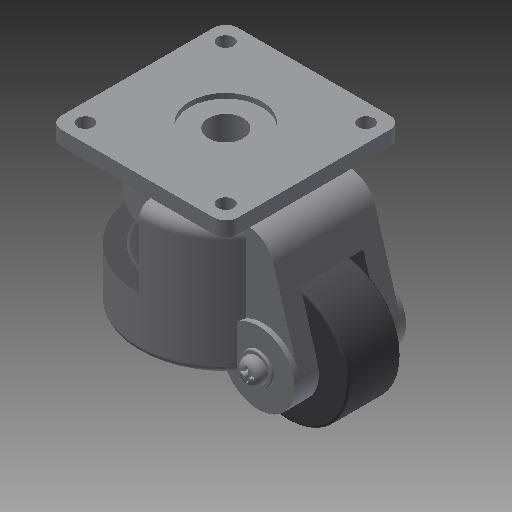
# Autodesk Inventor part: MayTec 1.45.80200.073_Locking castor 200kg, with plate
Saved by Autodesk Inventor 2018 (Build 220112000, 112)
## iProperties
Category: PARTsolutions
Company: MAYTEC
Created: 2012-11-13
Part Number: MayTec 1.45.80200.073_Locking castor 200kg, with plate
Catalog Web Link: www.cadenas.de
Description: Locking castor 200kg, with plate-Locking castor 200kg, with plate
Vendor: MAYTEC
Document SubType Name: Modeling
Designer: PARTuser1
Manufacturer: MAYTEC
Density: 1 g/cm^3
Material: Generic
Appearance: RGB(175.94999939203154,175.94999939203154,175.94999939203154)
PSOL_IDENT_0: {\\10.0.0.242\data_v9\23d-libs\maytec\maytec_3d\einbauzubehoer\rollen\feststell-rollen\1.45.80200.07
PSOL_IDENT_1: 3.prj},276 {VTYP=3D},{NB=MayTec 1.45.80200.073_Locking castor 200kg, with plate},{LINA=MayTec 1.45.8
PSOL_IDENT_2: 0200.073_Locking castor 200kg, with plate},{NN=Locking castor 200kg, with plate},{DATE=14.09.2010 08
PSOL_IDENT_3: :34:49},{GEOMDATE=28.01.2010 00:00:00},{VERSION=},{LINEID=10},{LINESUBID=-1},{WBVAR=}  {NB=MayTec 1.
PSOL_IDENT_4: 45.80200.073_Locking castor 200kg, with plate},{LINA=MayTec 1.45.80200.073_Locking castor 200kg, wit
PSOL_IDENT_5: h plate},{KT=DUMMY},{PARTNR=1.45.80200.073},{DESCRIPTION=Feststell-Rolle 200kg, mit Platte},{D=50.0}
PSOL_IDENT_6: ,{XTRANS=Locking castor 200kg, with plate}
CNS_NT: Locking castor 200kg, with plate
CNS_NB: MayTec 1.45.80200.073_Locking castor 200kg, with plate
CNS_NBSYN: MayTec $PARTNR._$XTRANS.
CNS_LINA: MayTec 1.45.80200.073_Locking castor 200kg, with plate
CNS_PARTNR: 1.45.80200.073
CNS_DESCRIPTION: Feststell-Rolle 200kg, mit Platte
CNS_D: 50.0
CNS_XTRANS: Locking castor 200kg, with plate
SUPPLIER: MAYTEC
ARTICLENO: MayTec 1.45.80200.073_Locking castor 200kg, with plate
BOMINFO: MayTec 1.45.80200.073_Locking castor 200kg, with plate
CREATOR: CADENAS GmbH
Title: MayTec 1.45.80200.073_Locking castor 200kg, with plate
Author: Cadenas PARTsolutions
Comments: Locking castor 200kg, with plate
Autodesk Inventor part; units mm, degrees
sketch "Sketch_2" plane through (0, 0, 0) normal (0, 1, 0) x (-1, 0, 0)
  line L0 (36.5, -31.5) -> (36.5, 31.5)
  arc A0 (36.5, 31.5) -> (31.5, 36.5) centre (31.5, 31.5) ccw
  line L1 (31.5, 36.5) -> (-31.5, 36.5)
  arc A1 (-31.5, 36.5) -> (-36.5, 31.5) centre (-31.5, 31.5) ccw
  line L2 (-36.5, 31.5) -> (-36.5, -31.5)
  arc A2 (-36.5, -31.5) -> (-31.5, -36.5) centre (-31.5, -31.5) ccw
  line L3 (-31.5, -36.5) -> (31.5, -36.5)
  arc A3 (31.5, -36.5) -> (36.5, -31.5) centre (31.5, -31.5) ccw
  circle A4 centre (-29, 29) radius 3.25
  circle A5 centre (-29, -29) radius 3.25
  circle A6 centre (29, 29) radius 3.25
  circle A7 centre (29, -29) radius 3.25
  constraints: 8 centre point, 8 end point, 8 point on circle
sketch "Sketch_1" plane through (0, 0, 0) normal (0, 0, 1) x (1, 0, 0)
  line L0 (0, -72) -> (0, -6)
  line L1 (0, -6) -> (29, -6)
  arc A0 (29, -6) -> (27.5, -7) centre (29.4232, -8.2598) ccw
  line L2 (27.5, -7) -> (17.5, -7)
  line L3 (17.5, -7) -> (17.5, -8)
  line L4 (17.5, -8) -> (28.5, -8)
  arc A1 (29, -8.5) -> (28.5, -8) centre (28.5, -8.5) ccw
  line L5 (29, -8.5) -> (29, -9.5)
  arc A2 (29, -9.5) -> (31, -11.5) centre (31, -9.5) ccw
  arc A3 (36, -16.5) -> (31, -11.5) centre (31, -16.5) ccw
  line L6 (36, -16.5) -> (36, -62)
  arc A4 (33, -65) -> (36, -62) centre (33, -62) ccw
  line L7 (33, -65) -> (30, -65)
  arc A5 (29, -64) -> (30, -65) centre (30, -64) ccw
  line L8 (29, -64) -> (29, -41)
  line L9 (29, -41) -> (28, -41)
  line L10 (28, -41) -> (28, -59)
  arc A6 (27.6154, -60.9231) -> (28, -59) centre (23, -59) ccw
  line L11 (27.6154, -60.9231) -> (24.2821, -68.9231)
  arc A7 (19.6667, -72) -> (24.2821, -68.9231) centre (19.6667, -67) ccw
  line L12 (19.6667, -72) -> (0, -72)
  line L13 (0, -72) -> (0, -6)
  constraints: 28 end point, 16 point on circle, 8 centre point
sketch "Sketch_3" plane through (0, 0, 0) normal (0, 0, 1) x (1, 0, 0)
  line L0 (14.7107, -52.434) -> (23.2335, -52.434)
  line L1 (23.2335, -52.434) -> (23.2335, -65)
  arc A0 (23.2335, -65) -> (50.8593, -53.6628) centre (36.5, -58) ccw
  line L2 (50.8593, -53.6628) -> (40.6951, -19.4721)
  arc A1 (40.6951, -19.4721) -> (31, -11.5) centre (29.9412, -22.669) ccw
  line L3 (31, -11.5) -> (14.7107, -11.5)
  line L4 (14.7107, -11.5) -> (14.7107, -52.434)
  constraints: 10 end point, 4 point on circle, 2 centre point
extrude "Extrusion1" add sketch "Sketch_3" along normal mid plane 42
revolve "Revolution1" add sketch "Sketch_1" angle 360 about axis through (0, -72, 0) along (0, -1, 0)
extrude "Extrusion2" add sketch "Sketch_2" against normal blind 6
sketch "Sketch_5" plane through (0, -72, 0) normal (0, 1, 0) x (1, 0, 0)
  arc A0 (9, -11) -> (11, -13) centre (11, -11) ccw
  line L0 (11, -13) -> (55, -13)
  line L1 (55, -13) -> (55, 13)
  line L2 (55, 13) -> (11, 13)
  arc A1 (11, 13) -> (9, 11) centre (11, 11) ccw
  line L3 (9, 11) -> (9, -11)
  constraints: 8 end point, 4 point on circle, 2 centre point
sketch "Sketch_4" plane through (0, 0, 0) normal (0, 0, 1) x (1, 0, 0)
  circle A0 centre (36.5, -58) radius 15
  constraints: 1 centre point
extrude "Extrusion3" add sketch "Sketch_4" along normal mid plane 46
extrude "Extrusion4" cut sketch "Sketch_5" along normal mid plane 84
sketch "Sketch_7" plane through (0, 0, 0) normal (0, 0, 1) x (1, 0, 0)
  circle A0 centre (36.5, -58) radius 5
  constraints: 1 centre point
extrude "Extrusion5" add sketch "Sketch_7" along normal mid plane 45
sketch "Sketch_6" plane through (36.5, 0, 0) normal (1, 0, 0) x (0, 0, -1)
  line L0 (50, -58) -> (-50, -58)
  line L1 (-12, -58) -> (-12, -48)
  line L2 (-12, -48) -> (-11, -48)
  line L3 (-11, -48) -> (-11, -34)
  arc A0 (-10, -33) -> (-11, -34) centre (-10, -34) ccw
  line L4 (-10, -33) -> (10, -33)
  arc A1 (11, -34) -> (10, -33) centre (10, -34) ccw
  line L5 (11, -34) -> (11, -48)
  line L6 (11, -48) -> (12, -48)
  line L7 (12, -48) -> (12, -58)
  line L8 (12, -58) -> (-12, -58)
  constraints: 18 end point, 4 point on circle, 2 centre point
sketch "Sketch_8" plane through (36.5, 0, 0) normal (1, 0, 0) x (0, 0, -1)
  line L0 (50, -58) -> (-50, -58)
  line L1 (-28, -58) -> (-28, -56)
  arc A0 (-25, -53) -> (-28, -56) centre (-25, -56) ccw
  line L2 (-25, -53) -> (-24, -53)
  line L3 (-24, -53) -> (-24, -52)
  arc A1 (-23.5, -51.5) -> (-24, -52) centre (-23.5, -52) ccw
  line L4 (-23.5, -51.5) -> (-23, -51.5)
  line L5 (-23, -51.5) -> (-23, -57)
  line L6 (-23, -57) -> (23, -57)
  line L7 (23, -57) -> (23, -51.5)
  line L8 (23, -51.5) -> (23.5, -51.5)
  arc A2 (24, -52) -> (23.5, -51.5) centre (23.5, -52) ccw
  line L9 (24, -52) -> (24, -53)
  line L10 (24, -53) -> (25, -53)
  arc A3 (28, -56) -> (25, -53) centre (25, -56) ccw
  line L11 (28, -56) -> (28, -58)
  line L12 (28, -58) -> (-28, -58)
  constraints: 26 end point, 8 point on circle, 4 centre point
revolve "Revolution2" add sketch "Sketch_8" angle 360 about axis through (36.5, -58, -50) along (0, 0, -1)
sketch "Sketch_9" plane through (36.5, -58, 28) normal (0, 0, 1) x (0, 1, 0)
  line L0 (-3, -0.5) -> (-1.5, -0.5)
  arc A0 (-0.5, -1.5) -> (-1.5, -0.5) centre (-1.5, -1.5) ccw
  line L1 (-0.5, -1.5) -> (-0.5, -3)
  line L2 (-0.5, -3) -> (0.5, -3)
  line L3 (0.5, -3) -> (0.5, -1.5)
  arc A1 (1.5, -0.5) -> (0.5, -1.5) centre (1.5, -1.5) ccw
  line L4 (1.5, -0.5) -> (3, -0.5)
  line L5 (3, -0.5) -> (3, 0.5)
  line L6 (3, 0.5) -> (1.5, 0.5)
  arc A2 (0.5, 1.5) -> (1.5, 0.5) centre (1.5, 1.5) ccw
  line L7 (0.5, 1.5) -> (0.5, 3)
  line L8 (0.5, 3) -> (-0.5, 3)
  line L9 (-0.5, 3) -> (-0.5, 1.5)
  arc A3 (-1.5, 0.5) -> (-0.5, 1.5) centre (-1.5, 1.5) ccw
  line L10 (-1.5, 0.5) -> (-3, 0.5)
  line L11 (-3, 0.5) -> (-3, -0.5)
  constraints: 24 end point, 8 point on circle, 4 centre point
extrude "Extrusion6" cut sketch "Sketch_9" along normal mid plane 6
sketch "Sketch_10" plane through (36.5, -58, -28) normal (0, 0, -1) x (0, 1, 0)
  line L0 (-3, -0.5) -> (-1.5, -0.5)
  arc A0 (-0.5, -1.5) -> (-1.5, -0.5) centre (-1.5, -1.5) ccw
  line L1 (-0.5, -1.5) -> (-0.5, -3)
  line L2 (-0.5, -3) -> (0.5, -3)
  line L3 (0.5, -3) -> (0.5, -1.5)
  arc A1 (1.5, -0.5) -> (0.5, -1.5) centre (1.5, -1.5) ccw
  line L4 (1.5, -0.5) -> (3, -0.5)
  line L5 (3, -0.5) -> (3, 0.5)
  line L6 (3, 0.5) -> (1.5, 0.5)
  arc A2 (0.5, 1.5) -> (1.5, 0.5) centre (1.5, 1.5) ccw
  line L7 (0.5, 1.5) -> (0.5, 3)
  line L8 (0.5, 3) -> (-0.5, 3)
  line L9 (-0.5, 3) -> (-0.5, 1.5)
  arc A3 (-1.5, 0.5) -> (-0.5, 1.5) centre (-1.5, 1.5) ccw
  line L10 (-1.5, 0.5) -> (-3, 0.5)
  line L11 (-3, 0.5) -> (-3, -0.5)
  constraints: 24 end point, 8 point on circle, 4 centre point
extrude "Extrusion7" cut sketch "Sketch_10" along normal mid plane 6
sketch "Sketch_11" plane through (0, -7, 0) normal (0, 1, 0) x (1, 0, 0)
  arc A0 (0, 36) -> (0, -36) centre (0, 0) ccw
  line L0 (0, -36) -> (0, -30)
  arc A1 (0, 30) -> (0, -30) centre (0, 0) ccw
  line L1 (0, 30) -> (0, 36)
  constraints: 4 end point, 4 point on circle, 2 centre point
extrude "Extrusion8" cut sketch "Sketch_11" against normal blind 36
sketch "Sketch_12" plane through (-30, 0, 0) normal (1, 0, 0) x (0, 0, -1)
  line L0 (-30, -25) -> (-30, -43)
  line L1 (-30, -43) -> (30, -43)
  line L2 (30, -43) -> (30, -25)
  line L3 (30, -25) -> (-30, -25)
  constraints: 8 end point
extrude "Extrusion9" cut sketch "Sketch_12" along normal blind 48
sketch "Sketch_13" plane through (0, -33, 0) normal (0, 1, 0) x (1, 0, 0)
  arc A0 (-24.5196, 4.8773) -> (-24.5196, -4.8773) centre (0, 0) ccw
  line L0 (-24.5196, -4.8773) -> (-17.324, -3.446)
  arc A1 (-17.324, -3.446) -> (-14.6866, -9.8133) centre (0, 0) ccw
  line L1 (-14.6866, -9.8133) -> (-20.7867, -13.8893)
  arc A2 (-20.7867, -13.8893) -> (-13.8893, -20.7867) centre (0, 0) ccw
  line L2 (-13.8893, -20.7867) -> (-9.8133, -14.6866)
  arc A3 (-9.8133, -14.6866) -> (-3.446, -17.324) centre (0, 0) ccw
  line L3 (-3.446, -17.324) -> (-4.8773, -24.5196)
  arc A4 (-4.8773, -24.5196) -> (4.8773, -24.5196) centre (0, 0) ccw
  line L4 (4.8773, -24.5196) -> (3.446, -17.324)
  arc A5 (3.446, -17.324) -> (9.8133, -14.6866) centre (0, 0) ccw
  line L5 (9.8133, -14.6866) -> (13.8893, -20.7867)
  arc A6 (13.8893, -20.7867) -> (20.7867, -13.8893) centre (0, 0) ccw
  line L6 (20.7867, -13.8893) -> (14.6866, -9.8133)
  arc A7 (14.6866, -9.8133) -> (17.324, -3.446) centre (0, 0) ccw
  line L7 (17.324, -3.446) -> (24.5196, -4.8773)
  arc A8 (24.5196, -4.8773) -> (24.5196, 4.8773) centre (0, 0) ccw
  line L8 (24.5196, 4.8773) -> (17.324, 3.446)
  arc A9 (17.324, 3.446) -> (14.6866, 9.8133) centre (0, 0) ccw
  line L9 (14.6866, 9.8133) -> (20.7867, 13.8893)
  arc A10 (20.7867, 13.8893) -> (13.8893, 20.7867) centre (0, 0) ccw
  line L10 (13.8893, 20.7867) -> (9.8133, 14.6866)
  arc A11 (9.8133, 14.6866) -> (3.446, 17.324) centre (0, 0) ccw
  line L11 (3.446, 17.324) -> (4.8773, 24.5196)
  arc A12 (4.8773, 24.5196) -> (-4.8773, 24.5196) centre (0, 0) ccw
  line L12 (-4.8773, 24.5196) -> (-3.446, 17.324)
  arc A13 (-3.446, 17.324) -> (-9.8133, 14.6866) centre (0, 0) ccw
  line L13 (-9.8133, 14.6866) -> (-13.8893, 20.7867)
  arc A14 (-13.8893, 20.7867) -> (-20.7867, 13.8893) centre (0, 0) ccw
  line L14 (-20.7867, 13.8893) -> (-14.6866, 9.8133)
  arc A15 (-14.6866, 9.8133) -> (-17.324, 3.446) centre (0, 0) ccw
  line L15 (-17.324, 3.446) -> (-24.5196, 4.8773)
  constraints: 32 end point, 32 point on circle, 16 centre point
extrude "Extrusion10" add sketch "Sketch_13" along normal blind 7
sketch "Sketch_14" plane through (0, -33, 0) normal (0, 1, 0) x (1, 0, 0)
  line L0 (-7, 4.0415) -> (-7, -4.0415)
  line L1 (-7, -4.0415) -> (0, -8.0829)
  line L2 (0, -8.0829) -> (7, -4.0415)
  line L3 (7, -4.0415) -> (7, 4.0415)
  line L4 (7, 4.0415) -> (0, 8.0829)
  line L5 (0, 8.0829) -> (-7, 4.0415)
  constraints: 12 end point
extrude "Extrusion11" add sketch "Sketch_14" against normal blind 8
sketch "Sketch_15" plane through (0, -49, 0) normal (0, 1, 0) x (1, 0, 0)
  circle A0 centre (0, 0) radius 5
  constraints: 1 centre point
extrude "Extrusion12" add sketch "Sketch_15" along normal blind 28
sketch "Sketch16" plane through (0, 0, 0) normal (0, 1, 0) x (1, 0, 0)
  point P0 (0, 0)
hole "Drilling 1" at (0, 0, 0) direction (0, -1, 0) diameter 14.5 depth 19
sketch "Sketch_17" plane through (0, 0, 0) normal (0, 1, 0) x (-1, 0, 0)
  circle A0 centre (0, 0) radius 15
  constraints: 1 centre point
extrude "Extrusion13" cut sketch "Sketch_17" against normal blind 2
revolve "Revolution3" add sketch "Sketch_6" angle 360 about axis through (36.5, -58, -50) along (0, 0, -1)
ref_plane "start_XY" through (0, 0, 0) normal (0, 1, 0) x (1, 0, 0)
ref_plane "start_YZ" through (0, 0, 0) normal (1, 0, 0) x (0, 0, -1)
ref_plane "start_ZX" through (0, 0, 0) normal (0, 0, -1) x (0, 1, 0)
body "Solid1"
